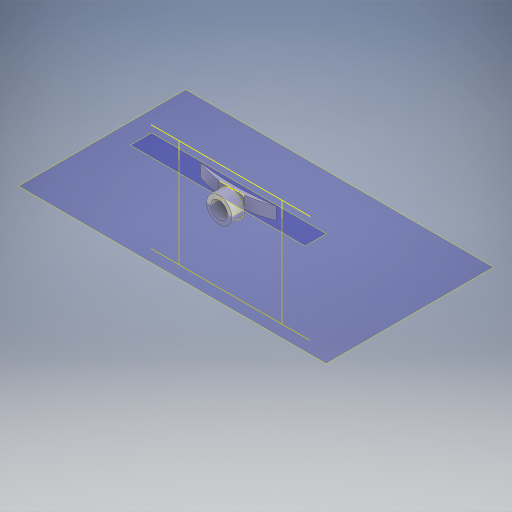
# Autodesk Inventor part: kick_panel
Saved by Autodesk Inventor 2023 (Build 270158000, 158)
## iProperties
Created: 2025-02-22
Part Number: kick_panel
Material: Типовые
Document SubType Name: Modeling
Designer: Ivan
Density: 1 g/cm^3
Appearance: По умолчанию
Author: Ivan
Autodesk Inventor part; units mm, degrees
ref_plane "YZ Plane" through (0, 0, 0) normal (1, 0, 0) x (0, 1, 0)
ref_plane "XZ Plane" through (0, 0, 0) normal (0, 1, 0) x (-1, 0, 0)
ref_plane "РабПлоскость1" through (0, 0, 0) normal (0, 0, 1) x (-1, 0, 0)
sketch "Эскиз1" plane through (0, 0, 0) normal (0, 0, 1) x (-1, 0, 0)
  circle A0 centre (6, 0) radius 3.75 projected
  line L0 (-30.812, 36.839) -> (43.1664, 36.839) projected
  line L1 (-30.812, -13.161) -> (43.1664, -13.161) projected
  circle A1 centre (6, 0) radius 6 projected
  line L2 (-17.8212, -13.161) -> (-17.8212, 36.839) projected
  line L3 (-17.8212, -13.161) -> (30.1756, -13.161) projected
  line L4 (30.1756, 36.839) -> (30.1756, -13.161) projected
  line L5 (-17.8212, 36.839) -> (30.1756, 36.839) projected
  point P0 (0, 0)
  constraints: 1 horizontal alignment
ref_plane "РабПлоскость2" through (-6, 0, 7.3222) normal (0, -1, 0) x (-1, 0, 0)
sketch "Эскиз2" plane through (-6, 0, 7.3222) normal (0, -1, 0) x (-1, 0, 0)
  line L0 (-3.75, 7.3222) -> (3.75, 7.3222) projected
  line L1 (0, -317.8644) -> (0, 181.8185)
  line L2 (3.75, 1.937) -> (-3.75, 1.937) construction
  arc A0 (3.75, 4.187) -> (-3.75, 4.187) centre (0, 4.187) ccw construction
  line L3 (3.835, 1.937) -> (-3.835, 1.937)
  line L4 (-3.835, 1.937) -> (-3.835, 8.137)
  line L5 (-3.835, 8.137) -> (3.835, 8.137)
  line L6 (3.835, 8.137) -> (3.835, 1.937)
  line L7 (6, 0) -> (6, 7.2771)
  line L8 (-6, 0) -> (-6, 7.3222)
  line L9 (5.89, 1.937) -> (-5.89, 1.937)
  line L10 (-5.89, 1.937) -> (-5.89, 8.137)
  line L11 (-5.89, 8.137) -> (5.89, 8.137) construction
  line L12 (5.89, 8.137) -> (5.89, 1.937)
  arc A1 (-36.812, 25.2187) -> (37.1664, 25.2187) centre (0.1772, 55.0189) ccw projected
  arc A2 (-17.4945, 10.9285) -> (17.5055, 10.7924) centre (0.4209, 117.7231) ccw
  line L13 (17.5055, 10.7924) -> (-17.4945, 10.9285) construction
  arc A3 (-36.812, 25.2187) -> (37.1664, 25.2187) centre (0.1772, 55.0189) ccw construction
  point P0 (0, 7.937)
  point P1 (0, 1.937)
  point P2 (0, 8.137)
  point P3 (5.89, 7.8636)
  point P4 (3.835, 7.6599)
  point P5 (0, 9.437)
  dimension "d1" = 7.5
  dimension "d2" = 7.67
  dimension "d3" = 0.2
  dimension "d4" = 12
  dimension "d5" = 11.78
  dimension "d8" = 1.3
  dimension "d9" = 35
  constraints: 24 end point, 9 point on circle, 5 midpoint, 4 parallel, 3 vertical, 2 centre point, 2 horizontal, 2 perpendicular, 1 point on line, 9 other
  measures "d1" distance of A0.end A0.start
  measures "d2" distance of L3.start L3.end
  measures "d3" distance from line of point (0, 7.937) L5
  measures "d4" distance between parallel lines of L8 L7
  measures "d5" distance of L10.end L11.end
  measures "d8" distance from line of point (0, 9.437) L5
  measures "d9" horizontal distance of L13.start L13.end
revolve "Вращение1" add sketch "Эскиз2" angle 360 about axis through (-6, 0, 325.1866) along (0, 0, -1) contours L6 A1 L12 L9
ref_plane "РабПлоскость3" through (-6, 5.89, 2.4219) normal (0, -1, 0) x (-1, 0, 0)
sketch "Эскиз5" plane through (-6, 5.89, 2.4219) normal (0, -1, 0) x (-1, 0, 0)
  line L0 (5.89, 2.9633) -> (-5.89, 2.9633) projected
  point P0 (-6, 2.4219)
  point P1 (0, 2.9633)
  constraints: 1 midpoint
sketch "Эскиз3" plane through (-6, 0, 7.3222) normal (0, -1, 0) x (-1, 0, 0)
  arc A0 (-17.4945, 10.9285) -> (17.5055, 10.7924) centre (0.4209, 117.7231) ccw projected
  arc A1 (-36.812, 25.2187) -> (37.1664, 25.2187) centre (0.1772, 55.0189) ccw projected
  line L0 (-5.89, 1.937) -> (-5.89, 8.137) projected
  line L1 (-3.835, 1.937) -> (-3.835, 8.137) projected
  line L2 (-3.835, 8.137) -> (3.835, 8.137) projected
  line L3 (5.89, 8.137) -> (5.89, 1.937) projected
  line L4 (5.89, 8.137) -> (5.89, 9.5744)
  line L5 (3.835, 7.6599) -> (-3.835, 7.6599) projected
  line L6 (5.89, 7.8636) -> (-5.89, 7.8636) projected
  line L7 (5.89, 7.8636) -> (-5.89, 7.8636) projected
  line L8 (-36.812, 7.3222) -> (37.1664, 7.3222) projected
  point P0 (-6, 7.3222)
  point P1 (5.89, 7.8636)
  point P2 (-5.5356, 7.8636)
  point P3 (-5.89, 7.3222)
  point P4 (5.89, 7.3222)
  point P5 (-3.4806, 7.6599)
  point P6 (-3.835, 7.6886)
  constraints: 2 end point, 1 point on circle, 1 vertical
extrude "Выдавливание1" add sketch "Эскиз3" against normal up to surface (5.89 mm away) contours A0 L4 L3 L6 A1 | A0 A1 L3 L4 | L6 L1 A1 | A1 L1 L8 L0 L6 | L3 L8 L1 L5 A1 | A1 L5 L1 L6 | A1 L5
